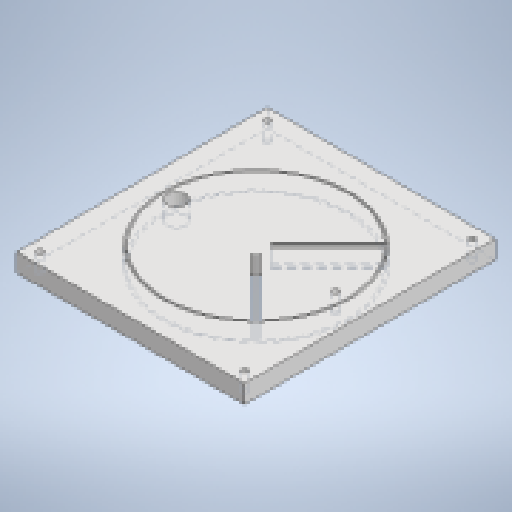
# Autodesk Inventor part: FlexK7V2
Saved by Autodesk Inventor 2023 (Build 270158000, 158)
## iProperties
Created: 2023-03-29
Part Number: FlexK7V2
Material: Generic
Document SubType Name: Modeling
Designer: Nathann
Density: 1 g/cm^3
Appearance: Default
Author: Nathann
Autodesk Inventor part; units mm, degrees
ref_plane "YZ Plane" through (0, 0, 0) normal (1, 0, 0) x (0, 1, 0)
ref_plane "XZ Plane" through (0, 0, 0) normal (0, 1, 0) x (-1, 0, 0)
ref_plane "XY Plane" through (0, 0, 0) normal (0, 0, 1) x (1, 0, 0)
sketch "Sketch1" plane through (0, 0, 0) normal (0, 1, 0) x (-1, 0, 0)
  line L0 (0, 0) -> (100, 0)
  line L1 (100, 0) -> (100, -110)
  line L2 (100, -110) -> (0, -110)
  line L3 (0, -110) -> (0, 0)
  line L4 (0, 0) -> (0, 0)
  line L5 (0, 0) -> (0, -150)
  line L6 (0, -150) -> (0, -150)
  line L7 (0, -150) -> (0, 0)
  line L8 (100, 0) -> (100, 0)
  line L9 (100, 0) -> (100, -150)
  line L10 (100, -150) -> (100, -150)
  line L11 (100, -150) -> (100, 0)
  point P0 (100, -110)
  point P1 (0, 0)
  point P2 (0, -110)
  dimension "d0" = 100
  dimension "d1" = 110
  dimension "d2" = 0
  dimension "d3" = 0
  dimension "d4" = 150
  dimension "d5" = 150
  constraints: 24 end point, 6 equal length, 3 horizontal, 3 perpendicular, 1 point on line
  measures "d0" distance of L0.start L0.end
  measures "d1" distance of L2.end L0.start
  measures "d2" distance of L9.end L10.end
  measures "d3" distance of L5.end L6.end
  measures "d4" distance of L4.end L5.end
  measures "d5" distance of L8.end L9.end
extrude "Extrusion1" add sketch "Sketch1" along normal blind 8
sketch "Sketch2" plane through (0, 8, 0) normal (0, 1, 0) x (1, 0, 0)
  circle A0 centre (-95, 5) radius 1.325
  line L0 (-100, 0) -> (0, 0) projected
  line L1 (-100, 110) -> (-100, 0) projected
  line L2 (-100, 55) -> (-85.0305, 55)
  line L3 (-50, 0) -> (-50, 9.4063)
  circle A1 centre (-95, 105) radius 1.325
  circle A2 centre (-5, 5) radius 1.325
  circle A3 centre (-5, 105) radius 1.325
  point P0 (0, 110)
  dimension "d118" = 5
  dimension "d119" = 5
  dimension "d120" = 2.65
  constraints: 4 centre point, 4 end point, 3 symmetric about line, 2 midpoint, 1 horizontal, 1 vertical, 3 other
  measures "d118" distance from line of L0 A0.centre
  measures "d119" distance from line of L1 A0.centre
  measures "d120" diameter of A0
extrude "Extrusion2" cut sketch "Sketch2" against normal blind 20
sketch "Sketch8" plane through (0, 8, 0) normal (0, 1, 0) x (1, 0, 0)
  line L0 (0, 0) -> (0, 110) projected
  arc A0 (-46.8357, 58.8714) -> (-46.1286, 58.1643) centre (-50, 55) ccw
  line L1 (-100, 0) -> (0, 0) projected
  line L2 (-55, 55) -> (-100, 55)
  line L3 (-100, 110) -> (-100, 0) projected
  line L4 (-50.2848, 59.9919) -> (-50.2848, 110)
  line L5 (0, 110) -> (-100, 110) projected
  circle A1 centre (-50, 55) radius 41
  circle A2 centre (-15, 55) radius 1.375
  circle A3 centre (-85, 55) radius 4
  line L6 (-50, 55) -> (-21.7157, 83.2843)
  line L7 (-46.8357, 58.8714) -> (-21.3643, 84.3428)
  line L8 (-46.1286, 58.1643) -> (-20.6572, 83.6357)
  line L9 (-47.688, 59.4333) -> (-22.7963, 84.325)
  line L10 (-45.5667, 57.312) -> (-20.675, 82.2037)
  arc A4 (-22.7963, 84.325) -> (-20.675, 82.2037) centre (-50, 55) ccw
  line L11 (-50, 55) -> (-21.7157, 26.7157)
  line L12 (-45.5667, 52.688) -> (-20.675, 27.7963)
  line L13 (-47.688, 50.5667) -> (-22.7963, 25.675)
  line L14 (-46.8357, 51.1286) -> (-21.3643, 25.6572)
  line L15 (-46.1286, 51.8357) -> (-20.6572, 26.3643)
  point P0 (-54.7697, 53.5)
  point P1 (-54.7697, 56.5)
  point P2 (-48.7848, 59.8501)
  point P3 (-21.3644, 27.0715)
  point P4 (-22.0715, 26.3644)
  dimension "d134" = 10
  dimension "d132" = 50
  dimension "d133" = 55
  dimension "d136" = 82
  dimension "d145" = 35
  dimension "d146" = 0
  dimension "d147" = 2.75
  dimension "d155" = 8
  dimension "d156" = 35
  dimension "d157" = 45
  dimension "d158" = 0.5
  dimension "d159" = 0.5
  dimension "d160" = 1
  dimension "d161" = 1
  dimension "d164" = 90
  constraints: 24 end point, 4 centre point, 4 parallel, 4 point on circle, 2 coincident, 2 point on line, 1 midpoint, 1 vertical, 27 other
  measures "d132" distance from line of L0 point (-50, 55)
  measures "d133" distance from line of point (-50, 55) L1
  measures "d136" diameter of A1
  measures "d145" distance of A2.centre point (-50, 55)
  measures "d146" vertical distance of point (-50, 55) A2.centre
  measures "d147" diameter of A2
  measures "d155" diameter of A3
  measures "d156" distance of point (-50, 55) A3.centre
  measures "d157" angle of L4 L6
  measures "d158" distance between parallel lines of L7 L6
  measures "d159" distance between parallel lines of L8 L6
  measures "d160" distance between parallel lines of L9 L7
  measures "d161" distance between parallel lines of L10 L8
extrude "Extrusion5" cut sketch "Sketch8" against normal blind 20 contours A1 L7 A0 L9 A4 L4 | L4 A4 L2 A1 | L2 A4 L14 A1 | A1 L15 A4 L10 A0 L8 | A3 L2 | L2 A3 | L13 A0 L14 A4 | L15 A0 L12 A4 | A2
sketch "Sketch9" plane through (0, 8, 0) normal (0, 1, 0) x (1, 0, 0)
  arc A0 (-22.7963, 84.325) -> (-22.7963, 25.675) centre (-50, 55) ccw projected
  line L0 (-90, 55) -> (-89, 55)
  line L1 (-89, 55) -> (-89, 13)
  line L2 (-89, 13) -> (-90, 13)
  line L3 (-90, 13) -> (-90, 55)
  line L4 (-90, 13) -> (-85, 13)
  line L5 (-85, 13) -> (-85, 3)
  line L6 (-85, 3) -> (-90, 3)
  line L7 (-90, 3) -> (-90, 13)
  line L8 (-85, 13) -> (-55, 13)
  line L9 (-55, 13) -> (-55, 12)
  line L10 (-55, 12) -> (-85, 12)
  line L11 (-85, 12) -> (-85, 13)
  line L12 (-85, 3) -> (-55, 3)
  line L13 (-55, 3) -> (-55, 4)
  line L14 (-55, 4) -> (-85, 4)
  line L15 (-85, 4) -> (-85, 3)
  line L16 (-100, 0) -> (0, 0) projected
  line L17 (-85, 5.5) -> (-55, 5.5)
  line L18 (-55, 5.5) -> (-55, 4.5)
  line L19 (-55, 4.5) -> (-85, 4.5)
  line L20 (-85, 4.5) -> (-85, 5.5)
  line L21 (-100, 0) -> (0, 0) projected
  line L22 (-48.4907, 0) -> (-63.4907, 0)
  line L23 (-63.4907, 0) -> (-63.4907, 4)
  line L24 (-63.4907, 4) -> (-48.4907, 4)
  line L25 (-48.4907, 4) -> (-48.4907, 0)
  line L26 (-55, 13) -> (-55, 14.306)
  arc A1 (-21.3643, 84.3428) -> (-21.3643, 25.6572) centre (-50, 55) ccw projected
  line L27 (-55, 12) -> (-55, 5.5)
  line L28 (-55, 4) -> (-55, 4.5)
  line L29 (-91, 55) -> (-100, 55)
  point P0 (-48.4907, 2)
  dimension "d166" = 1
  dimension "d167" = 1
  dimension "d168" = 1
  dimension "d169" = 30
  dimension "d170" = 10
  dimension "d171" = 3
  dimension "d172" = 5
  dimension "d173" = 6.5
  dimension "d174" = 1
  dimension "d175" = 0.5
  dimension "d176" = 30
  dimension "d177" = 15
  dimension "d178" = 4
  constraints: 56 end point, 12 parallel, 7 horizontal, 6 perpendicular, 4 point on line, 3 point on circle, 1 midpoint, 1 vertical
  measures "d166" distance between parallel lines of L8 L10
  measures "d167" distance between parallel lines of L14 L12
  measures "d168" distance between parallel lines of L3 L1
  measures "d169" distance of L9.end L10.end
  measures "d170" distance between parallel lines of L4 L6
  measures "d171" distance between parallel lines of L16 L6
  measures "d172" distance between parallel lines of L5 L7
  measures "d173" distance between parallel lines of L10 L17
  measures "d174" distance between parallel lines of L19 L17
  measures "d175" distance between parallel lines of L14 L19
  measures "d176" distance of L18.end L19.end
  measures "d177" distance from line of point (-48.491, 2) L23
  measures "d178" distance of L24.end L22.start
equation "\"d19\" = d18"
equation "\"d21\" = d22"
equation "\"BladeThickness\" = 1"
equation "\"NeckThickness\" = 1"
equation "\"d18\" = 45"
equation "\"d22\" = 47"
body "Solid1"
